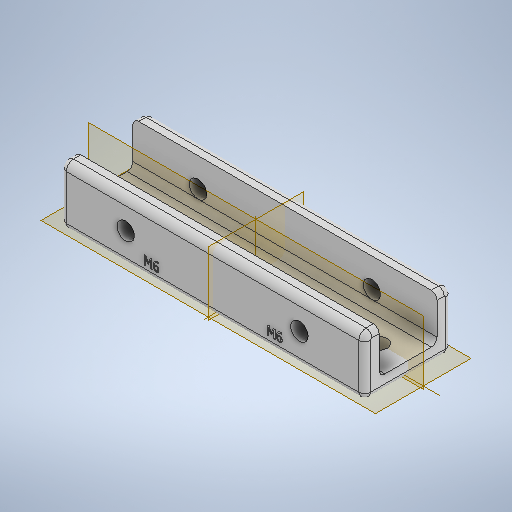
# Autodesk Inventor part: LaserMountRail
Saved by Autodesk Inventor 2025 (Build 290162000, 162)
## iProperties
Created: 2024-06-07
Part Number: LaserMountRail
Material: Generic
Document SubType Name: Modeling
Designer: mumin
Density: 1 g/cm^3
Appearance: Default
Author: mumin
Autodesk Inventor part; units mm, degrees
sketch "Sketch6" plane through (0, 0, 0) normal (1, 0, 0) x (0, 1, 0)
  line L0 (17.5, -15) -> (2, -15)
  line L1 (0, -13) -> (0, 13)
  line L2 (2, 15) -> (17.5, 15)
  line L3 (-4.6006, 0) -> (24.7042, 0) projected
  line L4 (20, 10) -> (7, 10)
  line L5 (5, 8) -> (5, -8)
  line L6 (7, -10) -> (20, -10)
  line L7 (20, -12.5) -> (20, -10)
  line L8 (20, 10) -> (20, 12.5)
  arc A0 (5, -8) -> (7, -10) centre (7, -8) ccw
  arc A1 (7, 10) -> (5, 8) centre (7, 8) ccw
  arc A2 (0, -13) -> (2, -15) centre (2, -13) ccw
  arc A3 (2, 15) -> (0, 13) centre (2, 13) ccw
  arc A4 (17.5, -15) -> (20, -12.5) centre (17.5, -12.5) ccw
  arc A5 (20, 12.5) -> (17.5, 15) centre (17.5, 12.5) ccw
  point P0 (0, 0)
  point P1 (20, -15)
  point P2 (0, -15)
  point P3 (0, 15)
  dimension "d35" = 20
  dimension "d36" = 30
  dimension "d37" = 5
  dimension "d38" = 2
  dimension "d39" = 2.5
  constraints: 16 end point, 12 point on circle, 12 tangent, 6 centre point, 6 point on line, 4 equal radius, 4 perpendicular, 1 collinear, 1 horizontal, 1 vertical, 3 other
  measures "d35" distance of point (20, -15) point (0, -15)
  measures "d36" distance of point (0, -15) point (0, 15)
  measures "d37" distance between parallel lines of L1 L5
  measures "d38" radius of A0
  measures "d39" radius of A4
extrude "Extrusion2" add sketch "Sketch6" along normal mid plane 105
fillet "Fillet2" radius 2 18 edges at (-52.5, 20, 11.25) (-52.5, 9.75, 15) (-52.5, 0.5858, 14.4142) (-52.5, 0, 0) (-52.5, 0.5858, -14.4142) (-52.5, 9.75, -15) (-52.5, 19.2678, -14.2678) (-52.5, 20, -11.25) (-52.5, 19.2678, 14.2678) (52.5, 19.2678, -14.2678) (52.5, 9.75, -15) (52.5, 0.5858, -14.4142) (52.5, 0, 0) (52.5, 0.5858, 14.4142) (52.5, 9.75, 15) (52.5, 19.2678, 14.2678) (52.5, 20, 11.25) (52.5, 20, -11.25)
sketch "Sketch7" plane through (-52.5, 5, 8) normal (0, 1, 0) x (1, 0, 0)
  point P0 (52.5, 8)
  point P1 (52.5, 8)
  constraints: 1 coincident
hole "Hole4" at (0, 5, 0) direction (0, -1, 0) diameter 6.35 end through all
sketch "Sketch8" plane through (-52.5, 5, 8) normal (0, 1, 0) x (1, 0, 0)
  line L0 (126, 8) -> (-21, 8) projected
  line L1 (52.5, 29) -> (52.5, -13) projected
  point P0 (52.5, 8)
  point P1 (94.75, 8)
  dimension "d57" = 42.25
  constraints: 1 point on line
  measures "d57" distance from line of L1 point (94.75, 8)
hole "Hole5" at (42.25, 5, 0) direction (0, -1, 0) diameter 6 end through all
sketch "Sketch9" plane through (-50.5, 17.5, 15) normal (0, 0, 1) x (1, 0, 0)
  line L0 (-23, -17.5) -> (124, -17.5) projected
  line L1 (50.5, 6.5) -> (50.5, -21.5) projected
  point P0 (50.5, -17.5)
  point P1 (80.5, -7.5)
  dimension "d65" = 10
  dimension "d66" = 30
  measures "d65" distance from line of L0 point (80.5, -7.5)
  measures "d66" distance from line of L1 point (80.5, -7.5)
hole "Hole6" at (30, 10, 15) direction (0, 0, -1) diameter 6 end through all
mirror "Mirror4" about plane through (0, 0, 0) normal (1, 0, 0) of "Hole6", "Hole5"
sketch "Sketch10" plane through (-50.5, 17.5, 15) normal (0, 0, 1) x (1, 0, 0)
  line L0 (26.6359, -11.3584) -> (32.1539, -11.3584) construction
  line L1 (32.1539, -11.3584) -> (32.1539, -14.5275) construction
  line L2 (32.1539, -14.5275) -> (26.6359, -14.5275) construction
  line L3 (26.6359, -14.5275) -> (26.6359, -11.3584) construction
  line L4 (69.1646, -11.0891) -> (74.6826, -11.0891) construction
  line L5 (74.6826, -11.0891) -> (74.6826, -14.2581) construction
  line L6 (74.6826, -14.2581) -> (69.1646, -14.2581) construction
  line L7 (69.1646, -14.2581) -> (69.1646, -11.0891) construction
  line L8 (29.5579, -14.4633) -> (29.1529, -14.4633)
  line L9 (29.1529, -14.4633) -> (29.1529, -11.8376)
  line L10 (29.1529, -11.8376) -> (28.3575, -13.6235)
  line L11 (28.3575, -13.6235) -> (28.1105, -13.6235)
  line L12 (28.1105, -13.6235) -> (27.3226, -11.8376)
  line L13 (27.3226, -11.8376) -> (27.3226, -14.4633)
  line L14 (27.3226, -14.4633) -> (26.9447, -14.4633)
  line L15 (26.9447, -14.4633) -> (26.9447, -11.4153)
  line L16 (26.9447, -11.4153) -> (27.498, -11.4153)
  line L17 (27.498, -11.4153) -> (28.2587, -13.1122)
  line L18 (28.2587, -13.1122) -> (28.9948, -11.4153)
  line L19 (28.9948, -11.4153) -> (29.5579, -11.4153)
  line L20 (29.5579, -11.4153) -> (29.5579, -14.4633)
  spline S0 degree 2 poles (32.0156, -13.4753) (32.0156, -13.7099) (31.86, -14.1076) (31.7291, -14.241) knots 0 0 0 1 2 2 2
  spline S1 degree 2 poles (31.7291, -14.241) (31.5932, -14.3817) (31.2524, -14.5275) (31.0474, -14.5275) knots 0 0 0 1 2 2 2
  spline S2 degree 2 poles (31.0474, -14.5275) (30.8424, -14.5275) (30.504, -14.3892) (30.3755, -14.2508) knots 0 0 0 1 2 2 2
  spline S3 degree 2 poles (30.3755, -14.2508) (30.2174, -14.0853) (30.0396, -13.5296) (30.0396, -13.1245) knots 0 0 0 1 2 2 2
  spline S4 degree 2 poles (30.0396, -13.1245) (30.0396, -12.7268) (30.2026, -12.0871) (30.373, -11.85) knots 0 0 0 1 2 2 2
  spline S5 degree 2 poles (30.373, -11.85) (30.5385, -11.6178) (31.0622, -11.3584) (31.4055, -11.3584) knots 0 0 0 1 2 2 2
  spline S6 degree 2 poles (31.4055, -11.3584) (31.5068, -11.3584) (31.6846, -11.3782) (31.7513, -11.4004) knots 0 0 0 1 2 2 2
  line L21 (31.7513, -11.4004) -> (31.7513, -11.7932)
  line L22 (31.7513, -11.7932) -> (31.734, -11.7932)
  spline S7 degree 2 poles (31.734, -11.7932) (31.6772, -11.7635) (31.4697, -11.7117) (31.3512, -11.7117) knots 0 0 0 1 2 2 2
  spline S8 degree 2 poles (31.3512, -11.7117) (30.9708, -11.7117) (30.504, -12.2254) (30.4595, -12.7293) knots 0 0 0 1 2 2 2
  spline S9 degree 2 poles (30.4595, -12.7293) (30.6052, -12.628) (30.9115, -12.5169) (31.0943, -12.5169) knots 0 0 0 1 2 2 2
  spline S10 degree 2 poles (31.0943, -12.5169) (31.2721, -12.5169) (31.5389, -12.5885) (31.6846, -12.6972) knots 0 0 0 1 2 2 2
  spline S11 degree 2 poles (31.6846, -12.6972) (31.8526, -12.8232) (32.0156, -13.2134) (32.0156, -13.4753) knots 0 0 0 1 2 2 2
  spline S12 degree 2 poles (31.6006, -13.4925) (31.6006, -13.3048) (31.5018, -13.0504) (31.3932, -12.9615) knots 0 0 0 1 2 2 2
  spline S13 degree 2 poles (31.3932, -12.9615) (31.3117, -12.8973) (31.1091, -12.8553) (31.0029, -12.8553) knots 0 0 0 1 2 2 2
  spline S14 degree 2 poles (31.0029, -12.8553) (30.8596, -12.8553) (30.5904, -12.9417) (30.4595, -13.0232) knots 0 0 0 1 2 2 2
  spline S15 degree 2 poles (30.4595, -13.0232) (30.457, -13.0677) (30.4521, -13.1517) (30.4521, -13.2159) knots 0 0 0 1 2 2 2
  spline S16 degree 2 poles (30.4521, -13.2159) (30.4521, -13.5321) (30.5756, -13.9199) (30.6695, -14.0211) knots 0 0 0 1 2 2 2
  spline S17 degree 2 poles (30.6695, -14.0211) (30.7559, -14.1175) (30.9436, -14.194) (31.0498, -14.194) knots 0 0 0 1 2 2 2
  spline S18 degree 2 poles (31.0498, -14.194) (31.2968, -14.194) (31.6006, -13.8433) (31.6006, -13.4925) knots 0 0 0 1 2 2 2
  line L23 (72.0866, -14.1939) -> (71.6815, -14.1939)
  line L24 (71.6815, -14.1939) -> (71.6815, -11.5683)
  line L25 (71.6815, -11.5683) -> (70.8862, -13.3541)
  line L26 (70.8862, -13.3541) -> (70.6392, -13.3541)
  line L27 (70.6392, -13.3541) -> (69.8512, -11.5683)
  line L28 (69.8512, -11.5683) -> (69.8512, -14.1939)
  line L29 (69.8512, -14.1939) -> (69.4733, -14.1939)
  line L30 (69.4733, -14.1939) -> (69.4733, -11.1459)
  line L31 (69.4733, -11.1459) -> (70.0266, -11.1459)
  line L32 (70.0266, -11.1459) -> (70.7874, -12.8428)
  line L33 (70.7874, -12.8428) -> (71.5234, -11.1459)
  line L34 (71.5234, -11.1459) -> (72.0866, -11.1459)
  line L35 (72.0866, -11.1459) -> (72.0866, -14.1939)
  spline S19 degree 2 poles (74.5443, -13.2059) (74.5443, -13.4406) (74.3887, -13.8382) (74.2577, -13.9716) knots 0 0 0 1 2 2 2
  spline S20 degree 2 poles (74.2577, -13.9716) (74.1219, -14.1124) (73.781, -14.2581) (73.576, -14.2581) knots 0 0 0 1 2 2 2
  spline S21 degree 2 poles (73.576, -14.2581) (73.371, -14.2581) (73.0326, -14.1198) (72.9042, -13.9815) knots 0 0 0 1 2 2 2
  spline S22 degree 2 poles (72.9042, -13.9815) (72.7461, -13.816) (72.5683, -13.2602) (72.5683, -12.8552) knots 0 0 0 1 2 2 2
  spline S23 degree 2 poles (72.5683, -12.8552) (72.5683, -12.4575) (72.7313, -11.8178) (72.9017, -11.5806) knots 0 0 0 1 2 2 2
  spline S24 degree 2 poles (72.9017, -11.5806) (73.0672, -11.3485) (73.5908, -11.0891) (73.9342, -11.0891) knots 0 0 0 1 2 2 2
  spline S25 degree 2 poles (73.9342, -11.0891) (74.0354, -11.0891) (74.2133, -11.1089) (74.28, -11.1311) knots 0 0 0 1 2 2 2
  line L36 (74.28, -11.1311) -> (74.28, -11.5238)
  line L37 (74.28, -11.5238) -> (74.2627, -11.5238)
  spline S26 degree 2 poles (74.2627, -11.5238) (74.2059, -11.4942) (73.9984, -11.4423) (73.8798, -11.4423) knots 0 0 0 1 2 2 2
  spline S27 degree 2 poles (73.8798, -11.4423) (73.4994, -11.4423) (73.0326, -11.9561) (72.9882, -12.46) knots 0 0 0 1 2 2 2
  spline S28 degree 2 poles (72.9882, -12.46) (73.1339, -12.3587) (73.4402, -12.2475) (73.6229, -12.2475) knots 0 0 0 1 2 2 2
  spline S29 degree 2 poles (73.6229, -12.2475) (73.8008, -12.2475) (74.0676, -12.3192) (74.2133, -12.4279) knots 0 0 0 1 2 2 2
  spline S30 degree 2 poles (74.2133, -12.4279) (74.3812, -12.5538) (74.5443, -12.9441) (74.5443, -13.2059) knots 0 0 0 1 2 2 2
  spline S31 degree 2 poles (74.1293, -13.2232) (74.1293, -13.0355) (74.0305, -12.7811) (73.9218, -12.6921) knots 0 0 0 1 2 2 2
  spline S32 degree 2 poles (73.9218, -12.6921) (73.8403, -12.6279) (73.6378, -12.5859) (73.5316, -12.5859) knots 0 0 0 1 2 2 2
  spline S33 degree 2 poles (73.5316, -12.5859) (73.3883, -12.5859) (73.1191, -12.6724) (72.9882, -12.7539) knots 0 0 0 1 2 2 2
  spline S34 degree 2 poles (72.9882, -12.7539) (72.9857, -12.7984) (72.9807, -12.8823) (72.9807, -12.9466) knots 0 0 0 1 2 2 2
  spline S35 degree 2 poles (72.9807, -12.9466) (72.9807, -13.2627) (73.1042, -13.6505) (73.1981, -13.7518) knots 0 0 0 1 2 2 2
  spline S36 degree 2 poles (73.1981, -13.7518) (73.2846, -13.8481) (73.4723, -13.9247) (73.5785, -13.9247) knots 0 0 0 1 2 2 2
  spline S37 degree 2 poles (73.5785, -13.9247) (73.8255, -13.9247) (74.1293, -13.5739) (74.1293, -13.2232) knots 0 0 0 1 2 2 2
  point P0 (50.5, -17.5)
  constraints: 4 other
emboss "Emboss3" sketch "Sketch10" operation cut depth 1.5 direction (0, 0, -1)
sketch "Sketch11" plane through (-52.5, 5, 8) normal (0, 1, 0) x (1, 0, 0)
  line L0 (45.4923, 4.1114) -> (59.4479, 4.1114) construction
  line L1 (59.4479, 4.1114) -> (59.4479, 0.2656) construction
  line L2 (59.4479, 0.2656) -> (45.4923, 0.2656) construction
  line L3 (45.4923, 0.2656) -> (45.4923, 4.1114) construction
  line L4 (92.093, 4.0604) -> (97.6111, 4.0604) construction
  line L5 (97.6111, 4.0604) -> (97.6111, 0.8914) construction
  line L6 (97.6111, 0.8914) -> (92.093, 0.8914) construction
  line L7 (92.093, 0.8914) -> (92.093, 4.0604) construction
  line L8 (7.3951, 4.2437) -> (12.9131, 4.2437) construction
  line L9 (12.9131, 4.2437) -> (12.9131, 1.0746) construction
  line L10 (12.9131, 1.0746) -> (7.3951, 1.0746) construction
  line L11 (7.3951, 1.0746) -> (7.3951, 4.2437) construction
  line L12 (10.3171, 1.1388) -> (9.912, 1.1388)
  line L13 (9.912, 1.1388) -> (9.912, 3.7645)
  line L14 (9.912, 3.7645) -> (9.1167, 1.9787)
  line L15 (9.1167, 1.9787) -> (8.8697, 1.9787)
  line L16 (8.8697, 1.9787) -> (8.0817, 3.7645)
  line L17 (8.0817, 3.7645) -> (8.0817, 1.1388)
  line L18 (8.0817, 1.1388) -> (7.7038, 1.1388)
  line L19 (7.7038, 1.1388) -> (7.7038, 4.1868)
  line L20 (7.7038, 4.1868) -> (8.2571, 4.1868)
  line L21 (8.2571, 4.1868) -> (9.0179, 2.4899)
  line L22 (9.0179, 2.4899) -> (9.7539, 4.1868)
  line L23 (9.7539, 4.1868) -> (10.3171, 4.1868)
  line L24 (10.3171, 4.1868) -> (10.3171, 1.1388)
  spline S0 degree 2 poles (12.7747, 2.1269) (12.7747, 1.8922) (12.6191, 1.4945) (12.4882, 1.3611) knots 0 0 0 1 2 2 2
  spline S1 degree 2 poles (12.4882, 1.3611) (12.3524, 1.2204) (12.0115, 1.0746) (11.8065, 1.0746) knots 0 0 0 1 2 2 2
  spline S2 degree 2 poles (11.8065, 1.0746) (11.6015, 1.0746) (11.2631, 1.2129) (11.1347, 1.3513) knots 0 0 0 1 2 2 2
  spline S3 degree 2 poles (11.1347, 1.3513) (10.9766, 1.5168) (10.7987, 2.0725) (10.7987, 2.4776) knots 0 0 0 1 2 2 2
  spline S4 degree 2 poles (10.7987, 2.4776) (10.7987, 2.8753) (10.9618, 3.515) (11.1322, 3.7521) knots 0 0 0 1 2 2 2
  spline S5 degree 2 poles (11.1322, 3.7521) (11.2977, 3.9843) (11.8213, 4.2437) (12.1647, 4.2437) knots 0 0 0 1 2 2 2
  spline S6 degree 2 poles (12.1647, 4.2437) (12.2659, 4.2437) (12.4438, 4.2239) (12.5105, 4.2017) knots 0 0 0 1 2 2 2
  line L25 (12.5105, 4.2017) -> (12.5105, 3.8089)
  line L26 (12.5105, 3.8089) -> (12.4932, 3.8089)
  spline S7 degree 2 poles (12.4932, 3.8089) (12.4364, 3.8386) (12.2289, 3.8904) (12.1103, 3.8904) knots 0 0 0 1 2 2 2
  spline S8 degree 2 poles (12.1103, 3.8904) (11.7299, 3.8904) (11.2631, 3.3767) (11.2186, 2.8728) knots 0 0 0 1 2 2 2
  spline S9 degree 2 poles (11.2186, 2.8728) (11.3644, 2.9741) (11.6706, 3.0852) (11.8534, 3.0852) knots 0 0 0 1 2 2 2
  spline S10 degree 2 poles (11.8534, 3.0852) (12.0313, 3.0852) (12.298, 3.0136) (12.4438, 2.9049) knots 0 0 0 1 2 2 2
  spline S11 degree 2 poles (12.4438, 2.9049) (12.6117, 2.7789) (12.7747, 2.3887) (12.7747, 2.1269) knots 0 0 0 1 2 2 2
  spline S12 degree 2 poles (12.3598, 2.1096) (12.3598, 2.2973) (12.261, 2.5517) (12.1523, 2.6406) knots 0 0 0 1 2 2 2
  spline S13 degree 2 poles (12.1523, 2.6406) (12.0708, 2.7048) (11.8683, 2.7468) (11.762, 2.7468) knots 0 0 0 1 2 2 2
  spline S14 degree 2 poles (11.762, 2.7468) (11.6188, 2.7468) (11.3495, 2.6604) (11.2186, 2.5789) knots 0 0 0 1 2 2 2
  spline S15 degree 2 poles (11.2186, 2.5789) (11.2162, 2.5344) (11.2112, 2.4504) (11.2112, 2.3862) knots 0 0 0 1 2 2 2
  spline S16 degree 2 poles (11.2112, 2.3862) (11.2112, 2.07) (11.3347, 1.6822) (11.4286, 1.581) knots 0 0 0 1 2 2 2
  spline S17 degree 2 poles (11.4286, 1.581) (11.515, 1.4846) (11.7028, 1.4081) (11.809, 1.4081) knots 0 0 0 1 2 2 2
  spline S18 degree 2 poles (11.809, 1.4081) (12.056, 1.4081) (12.3598, 1.7588) (12.3598, 2.1096) knots 0 0 0 1 2 2 2
  line L27 (47.4411, 0.9276) -> (45.9542, 0.9276)
  line L28 (45.9542, 0.9276) -> (45.9542, 1.2388)
  line L29 (45.9542, 1.2388) -> (46.5074, 1.2388)
  line L30 (46.5074, 1.2388) -> (46.5074, 3.2815)
  line L31 (46.5074, 3.2815) -> (45.9542, 3.2815)
  line L32 (45.9542, 3.2815) -> (45.9542, 3.5606)
  spline S19 degree 2 poles (45.9542, 3.5606) (46.2678, 3.5606) (46.5642, 3.7385) (46.584, 3.9855) knots 0 0 0 1 2 2 2
  line L33 (46.584, 3.9855) -> (46.9002, 3.9855)
  line L34 (46.9002, 3.9855) -> (46.9002, 1.2388)
  line L35 (46.9002, 1.2388) -> (47.4411, 1.2388)
  line L36 (47.4411, 1.2388) -> (47.4411, 0.9276)
  line L37 (49.2689, 4.1114) -> (48.0759, 0.2656)
  line L38 (48.0759, 0.2656) -> (47.7301, 0.2656)
  line L39 (47.7301, 0.2656) -> (48.9182, 4.1114)
  line L40 (48.9182, 4.1114) -> (49.2689, 4.1114)
  line L41 (51.566, 1.9749) -> (51.2029, 1.9749)
  line L42 (51.2029, 1.9749) -> (51.2029, 0.9276)
  line L43 (51.2029, 0.9276) -> (50.8102, 0.9276)
  line L44 (50.8102, 0.9276) -> (50.8102, 1.9749)
  line L45 (50.8102, 1.9749) -> (49.464, 1.9749)
  line L46 (49.464, 1.9749) -> (49.464, 2.4047)
  line L47 (49.464, 2.4047) -> (50.8275, 3.9756)
  line L48 (50.8275, 3.9756) -> (51.2029, 3.9756)
  line L49 (51.2029, 3.9756) -> (51.2029, 2.3034)
  line L50 (51.2029, 2.3034) -> (51.566, 2.3034)
  line L51 (51.566, 2.3034) -> (51.566, 1.9749)
  line L52 (50.8102, 2.3034) -> (50.8102, 3.4939)
  line L53 (50.8102, 3.4939) -> (49.7851, 2.3034)
  line L54 (49.7851, 2.3034) -> (50.8102, 2.3034)
  line L55 (52.349, 4.1114) -> (52.2601, 2.9258)
  line L56 (52.2601, 2.9258) -> (51.9909, 2.9258)
  line L57 (51.9909, 2.9258) -> (51.902, 4.1114)
  line L58 (51.902, 4.1114) -> (52.349, 4.1114)
  line L59 (53.1197, 4.1114) -> (53.0307, 2.9258)
  line L60 (53.0307, 2.9258) -> (52.7615, 2.9258)
  line L61 (52.7615, 2.9258) -> (52.6726, 4.1114)
  line L62 (52.6726, 4.1114) -> (53.1197, 4.1114)
  line L63 (54.6906, 2.0761) -> (53.5371, 2.0761)
  line L64 (53.5371, 2.0761) -> (53.5371, 2.4466)
  line L65 (53.5371, 2.4466) -> (54.6906, 2.4466)
  line L66 (54.6906, 2.4466) -> (54.6906, 2.0761)
  line L67 (56.9754, 0.9276) -> (55.0957, 0.9276)
  line L68 (55.0957, 0.9276) -> (55.0957, 1.3598)
  spline S20 degree 2 poles (55.0957, 1.3598) (55.2982, 1.55) (55.6588, 1.9032) (55.8317, 2.0934) knots 0 0 0 1 2 2 2
  spline S21 degree 2 poles (55.8317, 2.0934) (56.18, 2.4763) (56.4344, 2.9357) (56.4344, 3.1802) knots 0 0 0 1 2 2 2
  spline S22 degree 2 poles (56.4344, 3.1802) (56.4344, 3.3087) (56.3554, 3.5013) (56.2838, 3.5631) knots 0 0 0 1 2 2 2
  spline S23 degree 2 poles (56.2838, 3.5631) (56.2121, 3.6248) (56.0244, 3.6866) (55.9108, 3.6866) knots 0 0 0 1 2 2 2
  spline S24 degree 2 poles (55.9108, 3.6866) (55.8021, 3.6866) (55.5798, 3.6322) (55.4785, 3.5903) knots 0 0 0 1 2 2 2
  spline S25 degree 2 poles (55.4785, 3.5903) (55.3921, 3.5557) (55.2315, 3.4569) (55.1821, 3.4223) knots 0 0 0 1 2 2 2
  line L69 (55.1821, 3.4223) -> (55.1599, 3.4223)
  line L70 (55.1599, 3.4223) -> (55.1599, 3.857)
  spline S26 degree 2 poles (55.1599, 3.857) (55.2859, 3.9188) (55.7379, 4.0398) (55.9404, 4.0398) knots 0 0 0 1 2 2 2
  spline S27 degree 2 poles (55.9404, 4.0398) (56.3677, 4.0398) (56.8494, 3.5878) (56.8494, 3.2025) knots 0 0 0 1 2 2 2
  spline S28 degree 2 poles (56.8494, 3.2025) (56.8494, 3.0222) (56.7654, 2.7208) (56.6913, 2.5924) knots 0 0 0 1 2 2 2
  spline S29 degree 2 poles (56.6913, 2.5924) (56.6172, 2.459) (56.4023, 2.1972) (56.2838, 2.0712) knots 0 0 0 1 2 2 2
  spline S30 degree 2 poles (56.2838, 2.0712) (56.0911, 1.8612) (55.6193, 1.4117) (55.4785, 1.2808) knots 0 0 0 1 2 2 2
  line L71 (55.4785, 1.2808) -> (56.9754, 1.2808)
  line L72 (56.9754, 1.2808) -> (56.9754, 0.9276)
  spline S31 degree 2 poles (59.2799, 2.4516) (59.2799, 1.6315) (58.8032, 0.8634) (58.3067, 0.8634) knots 0 0 0 1 2 2 2
  spline S32 degree 2 poles (58.3067, 0.8634) (57.8028, 0.8634) (57.331, 1.6464) (57.331, 2.4491) knots 0 0 0 1 2 2 2
  spline S33 degree 2 poles (57.331, 2.4491) (57.331, 3.2741) (57.8078, 4.0373) (58.3067, 4.0373) knots 0 0 0 1 2 2 2
  spline S34 degree 2 poles (58.3067, 4.0373) (58.8081, 4.0373) (59.2799, 3.2469) (59.2799, 2.4516) knots 0 0 0 1 2 2 2
  spline S35 degree 2 poles (58.7562, 1.5229) (58.8155, 1.6735) (58.8649, 2.1379) (58.8649, 2.4516) knots 0 0 0 1 2 2 2
  spline S36 degree 2 poles (58.8649, 2.4516) (58.8649, 2.7653) (58.8155, 3.2272) (58.7538, 3.3828) knots 0 0 0 1 2 2 2
  spline S37 degree 2 poles (58.7538, 3.3828) (58.692, 3.5384) (58.4771, 3.6989) (58.3067, 3.6989) knots 0 0 0 1 2 2 2
  spline S38 degree 2 poles (58.3067, 3.6989) (58.1363, 3.6989) (57.9164, 3.5384) (57.8522, 3.3778) knots 0 0 0 1 2 2 2
  spline S39 degree 2 poles (57.8522, 3.3778) (57.7905, 3.2222) (57.746, 2.748) (57.746, 2.4491) knots 0 0 0 1 2 2 2
  spline S40 degree 2 poles (57.746, 2.4491) (57.746, 2.128) (57.7855, 1.6982) (57.8498, 1.5303) knots 0 0 0 1 2 2 2
  spline S41 degree 2 poles (57.8498, 1.5303) (57.909, 1.3722) (58.1289, 1.2018) (58.3067, 1.2018) knots 0 0 0 1 2 2 2
  spline S42 degree 2 poles (58.3067, 1.2018) (58.4747, 1.2018) (58.6945, 1.3623) (58.7562, 1.5229) knots 0 0 0 1 2 2 2
  line L73 (95.0151, 0.9556) -> (94.61, 0.9556)
  line L74 (94.61, 0.9556) -> (94.61, 3.5813)
  line L75 (94.61, 3.5813) -> (93.8146, 1.7954)
  line L76 (93.8146, 1.7954) -> (93.5676, 1.7954)
  line L77 (93.5676, 1.7954) -> (92.7797, 3.5813)
  line L78 (92.7797, 3.5813) -> (92.7797, 0.9556)
  line L79 (92.7797, 0.9556) -> (92.4018, 0.9556)
  line L80 (92.4018, 0.9556) -> (92.4018, 4.0036)
  line L81 (92.4018, 4.0036) -> (92.9551, 4.0036)
  line L82 (92.9551, 4.0036) -> (93.7158, 2.3067)
  line L83 (93.7158, 2.3067) -> (94.4519, 4.0036)
  line L84 (94.4519, 4.0036) -> (95.0151, 4.0036)
  line L85 (95.0151, 4.0036) -> (95.0151, 0.9556)
  spline S43 degree 2 poles (97.4727, 1.9436) (97.4727, 1.709) (97.3171, 1.3113) (97.1862, 1.1779) knots 0 0 0 1 2 2 2
  spline S44 degree 2 poles (97.1862, 1.1779) (97.0504, 1.0371) (96.7095, 0.8914) (96.5045, 0.8914) knots 0 0 0 1 2 2 2
  spline S45 degree 2 poles (96.5045, 0.8914) (96.2995, 0.8914) (95.9611, 1.0297) (95.8326, 1.168) knots 0 0 0 1 2 2 2
  spline S46 degree 2 poles (95.8326, 1.168) (95.6746, 1.3335) (95.4967, 1.8893) (95.4967, 2.2944) knots 0 0 0 1 2 2 2
  spline S47 degree 2 poles (95.4967, 2.2944) (95.4967, 2.692) (95.6597, 3.3318) (95.8302, 3.5689) knots 0 0 0 1 2 2 2
  spline S48 degree 2 poles (95.8302, 3.5689) (95.9957, 3.8011) (96.5193, 4.0604) (96.8626, 4.0604) knots 0 0 0 1 2 2 2
  spline S49 degree 2 poles (96.8626, 4.0604) (96.9639, 4.0604) (97.1418, 4.0407) (97.2084, 4.0184) knots 0 0 0 1 2 2 2
  line L86 (97.2084, 4.0184) -> (97.2084, 3.6257)
  line L87 (97.2084, 3.6257) -> (97.1912, 3.6257)
  spline S50 degree 2 poles (97.1912, 3.6257) (97.1343, 3.6554) (96.9269, 3.7072) (96.8083, 3.7072) knots 0 0 0 1 2 2 2
  spline S51 degree 2 poles (96.8083, 3.7072) (96.4279, 3.7072) (95.9611, 3.1935) (95.9166, 2.6896) knots 0 0 0 1 2 2 2
  spline S52 degree 2 poles (95.9166, 2.6896) (96.0624, 2.7908) (96.3686, 2.902) (96.5514, 2.902) knots 0 0 0 1 2 2 2
  spline S53 degree 2 poles (96.5514, 2.902) (96.7293, 2.902) (96.996, 2.8304) (97.1418, 2.7217) knots 0 0 0 1 2 2 2
  spline S54 degree 2 poles (97.1418, 2.7217) (97.3097, 2.5957) (97.4727, 2.2055) (97.4727, 1.9436) knots 0 0 0 1 2 2 2
  spline S55 degree 2 poles (97.0578, 1.9263) (97.0578, 2.1141) (96.959, 2.3685) (96.8503, 2.4574) knots 0 0 0 1 2 2 2
  spline S56 degree 2 poles (96.8503, 2.4574) (96.7688, 2.5216) (96.5662, 2.5636) (96.46, 2.5636) knots 0 0 0 1 2 2 2
  spline S57 degree 2 poles (96.46, 2.5636) (96.3168, 2.5636) (96.0475, 2.4772) (95.9166, 2.3956) knots 0 0 0 1 2 2 2
  spline S58 degree 2 poles (95.9166, 2.3956) (95.9142, 2.3512) (95.9092, 2.2672) (95.9092, 2.203) knots 0 0 0 1 2 2 2
  spline S59 degree 2 poles (95.9092, 2.203) (95.9092, 1.8868) (96.0327, 1.499) (96.1266, 1.3978) knots 0 0 0 1 2 2 2
  spline S60 degree 2 poles (96.1266, 1.3978) (96.213, 1.3014) (96.4008, 1.2249) (96.507, 1.2249) knots 0 0 0 1 2 2 2
  spline S61 degree 2 poles (96.507, 1.2249) (96.754, 1.2249) (97.0578, 1.5756) (97.0578, 1.9263) knots 0 0 0 1 2 2 2
  point P0 (52.5, 8)
  constraints: 6 other
emboss "Emboss4" sketch "Sketch11" operation cut depth 1.5 direction (0, -1, 0)
equation "\"d65\" = 0.5 * d35"
body "Solid2"
